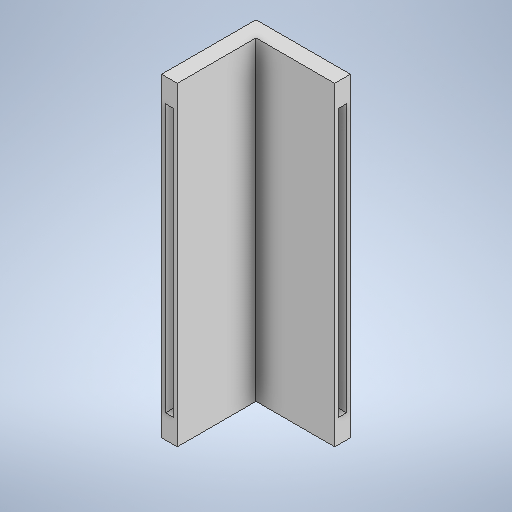
# Autodesk Inventor part: TSU_FF_Corner_Wall
Saved by Autodesk Inventor 2025.2 (Build 292293000, 293)
## iProperties
Created: 2025-01-07
Part Number: TSU_FF_Corner_Wall
Material: Generic
Document SubType Name: Modeling
Designer: Matt Tidd
Density: 1 g/cm^3
Appearance: Default
Author: Matt Tidd
Autodesk Inventor part; units mm, degrees
ref_plane "YZ Plane" through (0, 0, 0) normal (1, 0, 0) x (0, 1, 0)
ref_plane "XZ Plane" through (0, 0, 0) normal (0, 1, 0) x (-1, 0, 0)
ref_plane "XY Plane" through (0, 0, 0) normal (0, 0, 1) x (1, 0, 0)
sketch "Sketch1" plane through (0, 0, 0) normal (0, 1, 0) x (-1, 0, 0)
  line L0 (0, 0) -> (10, 0)
  line L1 (10, 0) -> (10, -60)
  line L2 (10, -60) -> (0, -60)
  line L3 (0, -60) -> (0, 0)
  line L4 (10, -60) -> (-50, -60)
  line L5 (-50, -60) -> (-50, -50)
  line L6 (-50, -50) -> (10, -50)
  line L7 (10, -50) -> (10, -60)
  point P0 (0, -50)
  point P1 (0, -60)
  dimension "d0" = 10
  dimension "d1" = 60
  dimension "d2" = 60
  dimension "d3" = 10
  constraints: 16 end point, 4 parallel, 2 horizontal, 2 perpendicular
  measures "d0" distance of L1.end L2.end
  measures "d1" distance of L0.end L1.end
  measures "d2" distance of L5.end L6.end
  measures "d3" distance of L4.end L5.end
extrude "Extrusion1" add sketch "Sketch1" along normal blind 200
sketch "Sketch2" plane through (-10, 0, 0) normal (0, 0, 1) x (1, 0, 0)
  line L0 (2.5, 15) -> (7.5, 15)
  line L1 (7.5, 15) -> (7.5, 185)
  line L2 (7.5, 185) -> (2.5, 185)
  line L3 (2.5, 185) -> (2.5, 15)
  point P0 (10, 0)
  dimension "d6" = 5
  dimension "d7" = 170
  constraints: 8 end point, 2 parallel, 1 horizontal, 1 perpendicular
  measures "d6" distance of L2.end L1.end
  measures "d7" distance of L1.end L0.end
extrude "Extrusion2" cut sketch "Sketch2" against normal blind 25
sketch "Sketch3" plane through (50, 0, -50) normal (1, 0, 0) x (0, 0, -1)
  line L0 (2.5, 15) -> (7.5, 15)
  line L1 (7.5, 15) -> (7.5, 185)
  line L2 (7.5, 185) -> (2.5, 185)
  line L3 (2.5, 185) -> (2.5, 15)
  point P0 (-50, 0)
  dimension "d10" = 5
  dimension "d11" = 170
  constraints: 8 end point, 2 parallel, 1 horizontal, 1 perpendicular
  measures "d10" distance of L2.end L1.end
  measures "d11" distance of L1.end L0.end
extrude "Extrusion3" cut sketch "Sketch3" against normal blind 25
body "Solid1"
